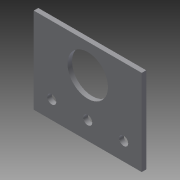
# Autodesk Inventor part: Elevator Shaft Mounts
Saved by Autodesk Inventor 2015 (Build 190159000, 159)
## iProperties
Created: 2015-02-11
Part Number: Elevator Shaft Mounts
Material: Generic
Document SubType Name: Modeling
Designer: chapale16
Density: 1 g/cm^3
Appearance: Default
Author: chapale16
Autodesk Inventor part; units mm, degrees
ref_plane "YZ Plane" through (0, 0, 0) normal (1, 0, 0) x (0, 1, 0)
ref_plane "XZ Plane" through (0, 0, 0) normal (0, 1, 0) x (-1, 0, 0)
ref_plane "XY Plane" through (0, 0, 0) normal (0, 0, 1) x (1, 0, 0)
sketch "Sketch1" plane through (0, 0, 0) normal (1, 0, 0) x (0, 1, 0)
  line L0 (0, 0) -> (-50.8, 0)
  line L1 (-50.8, 0) -> (-50.8, -25.4)
  line L2 (-50.8, -25.4) -> (0, -25.4)
  line L3 (0, -25.4) -> (0, 0)
  line L4 (-3.175, -3.175) -> (-47.625, -3.175)
  line L5 (-47.625, -3.175) -> (-47.625, -22.225)
  line L6 (-47.625, -22.225) -> (-3.175, -22.225)
  line L7 (-3.175, -22.225) -> (-3.175, -3.175)
  dimension "d0" = 50.8
  dimension "d1" = 25.4
  dimension "d2" = 3.175
  constraints: 16 end point, 4 parallel, 2 perpendicular, 1 horizontal, 3 other
  measures "d0" distance of L2.end L1.end
  measures "d1" distance of L1.end L0.end
  measures "d2" distance between parallel lines of L3 L7
extrude "Extrusion1" add sketch "Sketch1" along normal blind 127
sketch "Sketch2" plane through (0, -50.8, 0) normal (0, 0, 1) x (1, 0, 0)
  line L0 (0, 50.8) -> (0, 0) projected
  line L1 (0, 0) -> (127, 0) projected
  line L2 (127, 50.8) -> (127, 0) projected
  line L3 (0, 50.8) -> (127, 50.8) projected
  circle A0 centre (63.5, 6.0325) radius 3.175
  circle A1 centre (63.5, 33.3375) radius 6.35
  circle A2 centre (63.5, 33.3375) radius 14.2875
  circle A3 centre (63.5, 33.3375) radius 7.62
  circle A4 centre (63.5, 33.3375) radius 15.875
  line L4 (0, 47.625) -> (127, 47.625) projected
  dimension "d5" = 6.35
  dimension "d6" = 12.7
  dimension "d9" = 28.575
  dimension "d10" = 15.24
  dimension "d11" = 31.75
  dimension "d12" = 14.2875
  dimension "d13" = 16.51
  constraints: 5 centre point, 3 coincident
  measures "d5" diameter of A0
  measures "d6" diameter of A1
  measures "d9" diameter of A2
  measures "d10" diameter of A3
  measures "d11" diameter of A4
  measures "d12" distance from line of L4 A1.centre
extrude "Extrusion2" cut sketch "Sketch2" against normal blind 127 contours A2 | A0 | A1 | A3
sketch "Sketch3" plane through (0, -50.8, -25.4) normal (0, 0, -1) x (-1, 0, 0)
  circle A0 centre (-63.5, 33.3375) radius 14.2875 projected
  circle A1 centre (-63.5, 6.0325) radius 3.175 projected
  line L0 (0, 0) -> (0, 50.8) projected
  line L1 (0, 50.8) -> (-127, 50.8) projected
  line L2 (-127, 0) -> (-127, 50.8) projected
  line L3 (0, 0) -> (-127, 0) projected
  point P0 (-38.1, 6.0325)
  point P1 (-12.7, 6.0325)
  point P2 (-88.9, 6.0325)
  point P3 (-114.3, 6.0325)
  dimension "d16" = 25.4
  dimension "d17" = 25.4
  dimension "d18" = 25.4
  dimension "d19" = 25.4
  measures "d16" distance of A1.centre point (-88.9, 6.032)
  measures "d17" distance of point (-114.3, 6.032) point (-88.9, 6.032)
  measures "d18" distance of A1.centre point (-38.1, 6.032)
  measures "d19" distance of point (-12.7, 6.032) point (-38.1, 6.032)
hole "Hole1" at (38.1, -44.7675, -25.4) at (12.7, -44.7675, -25.4) at (88.9, -44.7675, -25.4) at (114.3, -44.7675, -25.4) direction (0, 0, 1) diameter 6.35 end through all
sketch "Sketch4" plane through (0, 0, 0) normal (-1, 0, 0) x (0, 0, 1)
  line L0 (0, 0) -> (-25.4, 0)
  line L1 (-25.4, 0) -> (-25.4, -101.6)
  line L2 (-25.4, -101.6) -> (0, -101.6)
  line L3 (0, -101.6) -> (0, 0)
  line L4 (-3.175, -98.425) -> (-22.225, -98.425)
  line L5 (-22.225, -98.425) -> (-22.225, -3.175)
  line L6 (-22.225, -3.175) -> (-3.175, -3.175)
  line L7 (-3.175, -3.175) -> (-3.175, -98.425)
  line L8 (-3.175, -47.625) -> (-3.175, -3.175) projected
  line L9 (-22.225, -61.2712) -> (-3.175, -61.2712)
  line L10 (-3.175, -61.2712) -> (-3.175, -33.0722)
  line L11 (-3.175, -33.0722) -> (-22.225, -33.0722)
  line L12 (-22.225, -33.0722) -> (-22.225, -61.2712)
  line L13 (-22.225, -3.175) -> (-3.175, -3.175) projected
  line L14 (-3.175, -3.175) -> (-3.175, -47.625) projected
  line L15 (-3.175, -47.625) -> (-22.225, -47.625) projected
  line L16 (-22.225, -47.625) -> (-22.225, -3.175) projected
  line L17 (0, 0) -> (0, -50.8) projected
  line L18 (-25.4, 0) -> (0, 0) projected
  line L19 (-25.4, -50.8) -> (-25.4, 0) projected
  line L20 (0, -50.8) -> (-25.4, -50.8) projected
  line L21 (-25.4, -50.8) -> (-22.225, -50.8)
  line L22 (0, -50.8) -> (-25.4, -50.8) projected
  line L23 (-3.175, -50.8) -> (0, -50.8)
  dimension "d27" = 25.4
  dimension "d28" = 101.6
  dimension "d29" = 3.175
  constraints: 28 end point, 6 parallel, 6 point on line, 3 perpendicular, 2 horizontal, 1 collinear, 3 other
  measures "d27" distance of L2.end L1.end
  measures "d28" distance of L1.end L0.end
  measures "d29" distance between parallel lines of L2 L4
extrude "Extrusion3" cut sketch "Sketch4" against normal blind 127 contours L20 L5 L15 L7 | L7 L9 L5 L20 | L15 L5 L11 L7
extrude "Extrusion4" add sketch "Sketch4" against normal blind 127 contours L3 L2 L1 L20 L5 L4 L7
sketch "Sketch5" plane through (127, 0, -25.4) normal (0, 0, -1) x (-1, 0, 0)
  line L0 (-34.6309, 15.7259) -> (-18.4019, -170.3675)
  line L1 (-18.4019, -170.3675) -> (166.6096, -150.8926)
  line L2 (166.6096, -150.8926) -> (166.6096, -41.3464)
  line L3 (166.6096, -41.3464) -> (138.7497, 15.7259)
  line L4 (138.7497, 15.7259) -> (-34.6309, 15.7259)
  point P0 (127, 0)
  constraints: 10 end point, 1 perpendicular, 1 vertical
extrude "Extrusion5" cut sketch "Sketch5" against normal blind 22.225
sketch "Sketch6" plane through (0, 0, 0) normal (0, 0, 1) x (1, 0, 0)
  circle A0 centre (12.7, -44.7675) radius 3.175 projected
  line L0 (12.7, -44.7675) -> (0, -44.7675)
  line L1 (0, 0) -> (0, -101.6) projected
  line L2 (0, -44.7675) -> (0, -57.4675)
  line L3 (0, -57.4675) -> (127, -57.4675)
  line L4 (127, 0) -> (127, -101.6) projected
  line L5 (12.7, -44.7675) -> (127, -44.7675)
  line L6 (127, -44.7675) -> (127, -57.4675)
  line L7 (127, -57.4675) -> (144.4596, -106.2687)
  line L8 (144.4596, -106.2687) -> (111.8065, -115.7811)
  line L9 (111.8065, -115.7811) -> (9.525, -135.9925)
  line L10 (9.525, -135.9925) -> (-52.3397, -101.6)
  line L11 (-52.3397, -101.6) -> (0, -57.4675)
  dimension "d36" = 12.7
  dimension "d37" = 12.7
  constraints: 20 end point, 5 point on line, 1 collinear, 1 perpendicular
  measures "d36" distance of L0.start L0.end
  measures "d37" distance of L0.end L2.end
extrude "Extrusion6" cut sketch "Sketch6" against normal blind 22.225 contours L7 L8 L9 L10 L11 L3
sketch "Sketch7" plane through (0, -57.4675, 0) normal (0, -1, 0) x (1, 0, 0)
  line L0 (127, -3.175) -> (127, 0)
  line L1 (0, 0) -> (127, 0) projected
  line L2 (127, 0) -> (0, 0)
  line L3 (0, 0) -> (0, -3.175)
  line L4 (0, -3.175) -> (127, -3.175)
  line L5 (127, -3.175) -> (0, -3.175) projected
  constraints: 8 end point, 3 perpendicular, 1 collinear
sketch "Sketch8" plane through (0, 0, 0) normal (0, 1, 0) x (1, 0, 0)
  line L0 (0, 0) -> (0, 3.175)
  line L1 (0, 3.175) -> (127, 3.175)
  line L2 (127, 3.175) -> (127, 0)
  line L3 (127, 0) -> (0, 0)
  constraints: 8 end point, 3 perpendicular, 1 vertical
extrude "Extrusion8" add sketch "Sketch8" along normal blind 3.1623
sketch "Sketch9" plane through (127, 0, 0) normal (1, 0, 0) x (0, 0, -1)
  line L0 (0, 3.1623) -> (3.175, 3.1623)
  line L1 (3.175, 3.1623) -> (0, 3.1623) projected
  line L2 (3.175, 3.1623) -> (3.175, -57.4675)
  line L3 (3.175, -57.4675) -> (0, -57.4675)
  line L4 (0, -57.4675) -> (3.175, -57.4675) projected
  line L5 (0, -57.4675) -> (0, 3.1623)
  point P0 (0, 0)
  constraints: 8 end point, 3 equal length, 1 perpendicular
extrude "Extrusion9" cut sketch "Sketch9" against normal blind 25.4
sketch "Sketch10" plane through (0, 0, 0) normal (-1, 0, 0) x (0, 0, 1)
  line L0 (0, 3.1623) -> (0, -57.4675)
  line L1 (0, -57.4675) -> (-3.175, -57.4675)
  line L2 (-3.175, -57.4675) -> (-3.175, 3.1623)
  line L3 (-3.175, 3.1623) -> (-3.175, -57.4675) projected
  line L4 (-3.175, 3.1623) -> (0, 3.1623)
  point P0 (0, 0)
  constraints: 8 end point, 2 perpendicular, 1 collinear, 1 vertical
extrude "Extrusion10" cut sketch "Sketch10" against normal blind 25.4
body "Solid1"
